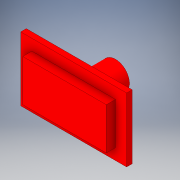
# Autodesk Inventor part: boton2
Saved by Autodesk Inventor 2019 (Build 230136000, 136)
## iProperties
Created: 2019-02-27
Part Number: boton2
Material: Genérico
Document SubType Name: Modeling
Designer: flakt
Density: 1 g/cm^3
Appearance: Valor por defecto
Author: flakt
Autodesk Inventor part; units mm, degrees
ref_plane "YZ Plane" through (0, 0, 0) normal (1, 0, 0) x (0, 1, 0)
ref_plane "XZ Plane" through (0, 0, 0) normal (0, 1, 0) x (-1, 0, 0)
ref_plane "XY Plane" through (0, 0, 0) normal (0, 0, 1) x (1, 0, 0)
sketch "Boceto1" plane through (0, 0, 0) normal (0, 0, 1) x (1, 0, 0)
  line L0 (-0.2897, 0) -> (29.7103, 0)
  line L1 (29.7103, 0) -> (29.7103, -15)
  line L2 (29.7103, -15) -> (-0.2897, -15)
  line L3 (-0.2897, -15) -> (-0.2897, 0)
  point P0 (0, 0)
  dimension "d0" = 30
  dimension "d1" = 15
  constraints: 8 end point, 2 parallel, 1 horizontal, 1 perpendicular
  measures "d0" distance of L1.end L2.end
  measures "d1" distance of L0.end L1.end
extrude "Extrusión1" add sketch "Boceto1" along normal blind 3.3
sketch "Boceto2" plane through (0, 0, 0) normal (0, 0, -1) x (-1, 0, 0)
  line L0 (-29.7103, -15) -> (0.2897, -15) projected
  line L1 (0.2897, 0) -> (-29.7103, 0) projected
  line L2 (-29.7103, 0) -> (-29.7103, -15) projected
  line L3 (-29.7103, -15) -> (0.2897, -15) projected
  line L4 (0.2897, -15) -> (0.2897, 0) projected
  line L5 (4.2897, 4) -> (-33.7103, 4)
  line L6 (-33.7103, 4) -> (-33.7103, -19)
  line L7 (-33.7103, -19) -> (4.2897, -19)
  line L8 (4.2897, -19) -> (4.2897, 4)
  point P0 (0, 0)
  dimension "d4" = 4
  constraints: 8 end point, 3 other
  measures "d4" distance between parallel lines of L4 L8
extrude "Extrusión2" add sketch "Boceto2" along normal blind 2 contours L2 L1 L4 L0 | L8 L7 L6 L5
sketch "Boceto3" plane through (0, 0, -2) normal (0, 0, -1) x (-1, 0, 0)
  line L0 (4.2897, 4) -> (-33.7103, 4) projected
  line L1 (-14.7103, 4) -> (-14.7103, -19)
  line L2 (-33.7103, -19) -> (4.2897, -19) projected
  circle A0 centre (-14.7103, -7.5) radius 5
  point P0 (0, 0)
  dimension "d7" = 10
  constraints: 3 midpoint, 2 end point, 1 centre point
  measures "d7" diameter of A0
extrude "Extrusión3" add sketch "Boceto3" along normal blind 13
